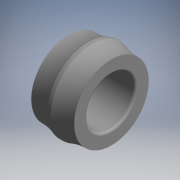
# Autodesk Inventor part: 22205/20 E_ir
Saved by Autodesk Inventor 2017.3 (Build 213256000, 256)
## iProperties
Part Number: 22205/20 E_ir
Material: Generic
Catalog Web Link: www.cadenas.de
Description: BS2_001-Spherical roller bearings
Vendor: SKF
Document SubType Name: Modeling
Designer: partserver
Manufacturer: SKF
Mass: 9.13352 g
Surface Area: 38.548 cm^2
Volume: 9.13352 cm^3
Density: 1 g/cm^3
Appearance: PSOLRGB-175-175-175
Category: PARTsolutions
Company: SKF
Title: 22205/20 E_ir
Author: Cadenas PARTsolutions
Comments: Spherical roller bearings
PSOL_IDENT_0: {$CADENAS_DATA\23d-libs\skf\bearings_units_and_housings\roller_bearings\spherical_roller_bearings\pa
PSOL_IDENT_1: rts\bs2_001_ir.prj},171 {VTYP=3D},{NB=22205/20 E_ir},{LINA=22205/20 E_ir},{NN=BS2_001},{DATE=23.12.2
PSOL_IDENT_2: 020 11:58:30},{GEOMDATE=25.11.2020 12:50:20},{VERSION=},{LINEID=460970},{WBVAR=},{WBNUMERIC=}  {NB=2
PSOL_IDENT_3: 2205/20 E_ir},{LINA=22205/20 E_ir},{KT=DUMMY},{DESIGNATION=22205/20 E},{VARIANT=CE1W33},{DESIGNX=Cyl
PSOL_IDENT_4: indrical bore},{SEAL=No seals},{SALG=NO},{BORE=20.000},{DD=20.000},{DD1=MIN},{D=52.000},{B=18.000},{
PSOL_IDENT_5: DD2=31.300},{DD3=MIN},{D1=44.200},{B1=MIN},{B2=MIN},{B4=MIN},{B5=MIN},{BB=3.700},{K=2.000},{R12=1.00
PSOL_IDENT_6: 0},{G=},{G1=MIN},{TB=MIN},{ALPHA=12.8333},{R34=MIN},{PITCH=39.459},{DW=7.130},{LW=6.600},{DDAMIN=25.
PSOL_IDENT_7: 600},{DDAMAX=MIN},{DBMIN=MIN},{DAMAX=46.400},{BAMIN=MIN},{RAMAX=1.000},{LOAD1=49.900},{LOAD2=44.000}
PSOL_IDENT_8: ,{LOAD3=4.750},{SPEED1=13000},{SPEED2=17000},{PRA=},{PLA=},{Z=15.000},{II=2.000},{MASS=0.280},{MASS2=
PSOL_IDENT_9: MIN},{SLEEVE=},{POPULAR=},{BEARING=22205/20 E},{PPATH=parts/bs2_001_asmtpl.prj},{RAMAXX=1},{EE=0.35}
PSOL_IDENT_10: ,{Y0=1.8},{R12X=1},{Y2=2.9},{ALPHAX=12.83333},{Y1=1.9},{DD1X=},{B1X=},{SLEEVEX=},{ALPHAXX=},{B2X=},{
PSOL_IDENT_11: SUPRESSED=},{BBALG=3.700},{KALG=2.000},{DESIGN=CB}
NB: 22205/20 E_ir
NN: BS2_001
NT: Spherical roller bearings
NBSYN: $DESIGNATION._ir
LINA: 22205/20 E_ir
CATALOG: SKF
DESIGNATION: 22205/20 E
VARIANT: CE1W33
DESIGNX: Cylindrical bore
SEAL: No seals
BORE: 20
DD: 20
DD1: 0
D: 52
B: 18
DD2: 31.3
DD3: 0
D1: 44.2
B1: 0
B2: 0
B4: 0
B5: 0
BB: 3.7
K: 2
R12: 1
G1: 0
TB: 0
ALPHA: 12.8333
R34: 0
PITCH: 39.459
DW: 7.13
LW: 6.6
DDAMIN: 25.6
DDAMAX: 0
DBMIN: 0
DAMAX: 46.4
BAMIN: 0
RAMAX: 1
LOAD1: 49.9
LOAD2: 44
LOAD3: 4.75
SPEED1: 13000
SPEED2: 17000
Z: 15
II: 2
MASS: 0.28
MASS2: 0
BEARING: 22205/20 E
PPATH: parts/bs2_001_asmtpl.prj
RAMAXX: 1
EE: 0.35
Y0: 1.8
R12X: 1
Y2: 2.9
ALPHAX: 12.83333
Y1: 1.9
SUPPLIER: SKF
ARTICLENO: 22205/20 E_ir
BOMINFO: 22205/20 E_ir
CREATOR: CADENAS GmbH
Autodesk Inventor part; units mm, degrees
sketch "Sketch_1" plane through (0, 0, 0) normal (0, 0, 1) x (1, 0, 0)
  line L0 (18, 0) -> (-18, 0)
  arc A0 (0, 11) -> (1, 10) centre (1, 11) ccw
  line L1 (1, 10) -> (17, 10)
  arc A1 (17, 10) -> (18, 11) centre (17, 11) ccw
  line L2 (18, 11) -> (18, 15.65)
  arc A2 (15.289, 15.7632) -> (18, 15.65) centre (17.3933, 33.6398) ccw
  arc A3 (9.7224, 17.0927) -> (15.289, 15.7632) centre (17.8763, 38.9136) ccw
  line L3 (9.7224, 17.0927) -> (8.2776, 17.0927)
  arc A4 (2.711, 15.7632) -> (8.2776, 17.0927) centre (0.1237, 38.9136) ccw
  arc A5 (0, 15.65) -> (2.711, 15.7632) centre (0.6067, 33.6398) ccw
  line L4 (0, 15.65) -> (0, 11)
  constraints: 12 point on circle, 10 end point, 6 centre point
revolve "Revolution1" add sketch "Sketch_1" angle 360 about axis through (18, 0, 0) along (1, 0, 0)
ref_plane "NO_GEO_XY" through (0, 0, 0) normal (1, 0, 0) x (0, 0, -1)
ref_plane "NO_GEO_YZ" through (0, 0, 0) normal (0, 0, -1) x (0, 1, 0)
ref_plane "NO_GEO_ZX" through (0, 0, 0) normal (0, 1, 0) x (1, 0, 0)
ref_plane "ir_XY" through (0, 0, 0) normal (0, 0, 1) x (1, 0, 0)
ref_plane "ir_YZ" through (0, 0, 0) normal (1, 0, 0) x (0, 1, 0)
ref_plane "ir_ZX" through (0, 0, 0) normal (0, 1, 0) x (0, 0, 1)
body "Solid1"
